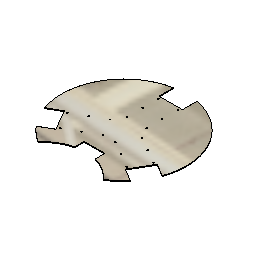
BaseChapaBaixo (Autodesk Fusion 360 design; units mm, degrees)
Autodesk Fusion 360 part; units mm, degrees
note: some values were not read from the file. Set by a fixed rule: which sketch regions a step uses.
sketch "Sketch1" plane through (0, 0, 0) normal (0, 1, 0) x (1, 0, 0)
  circle A0 centre (0, 0) radius 240
  line L0 (0, 0) -> (-207.8461, -120)
  line L1 (0, 0) -> (240, 0) construction
  line L2 (0, 0) -> (207.8461, -120)
  line L3 (0, 0) -> (240, 0) construction
  line L4 (0, 0) -> (0, 240)
  line L5 (0, 240) -> (0, 180)
  line L6 (0, 180) -> (-45, 180)
  line L7 (0, 180) -> (45, 180)
  line L8 (45, 180) -> (45, 235.7435)
  line L9 (-45, 180) -> (-45, 179.9979)
  line L10 (-45, 179.9979) -> (-45, 235.7435)
  line L11 (-133.3828, -128.9701) -> (-181.6599, -156.8429)
  line L12 (-155.8846, -90) -> (-133.3846, -128.9711)
  line L13 (-155.8846, -90) -> (-178.3846, -51.0289)
  line L14 (-178.3846, -51.0289) -> (-226.6599, -78.9006)
  line L15 (178.3828, -51.0278) -> (226.6599, -78.9006)
  line L16 (155.8846, -90) -> (178.3846, -51.0289)
  line L17 (155.8846, -90) -> (133.3846, -128.9711)
  line L18 (133.3846, -128.9711) -> (181.6599, -156.8429)
  line L19 (0, 180) -> (-37.5, 180)
  line L20 (-37.5, 180) -> (-37.5, 169.5)
  circle A1 centre (-37.5, 169.5) radius 2.5
  line L21 (-37.5, 169.5) -> (-37.5, 109.5)
  line L22 (-37.5, 109.5) -> (-37.5, 49.5)
  circle A2 centre (-37.5, 109.5) radius 2.5
  circle A3 centre (-37.5, 49.5) radius 2.5
  line L23 (37.5, 109.5) -> (37.5, 49.5)
  circle A4 centre (37.5, 49.5) radius 2.5
  circle A5 centre (37.5, 109.5) radius 2.5
  line L24 (37.5, 169.5) -> (37.5, 109.5)
  circle A6 centre (37.5, 169.5) radius 2.5
  line L25 (37.5, 180) -> (37.5, 169.5)
  circle A7 centre (-165.5413, -52.274) radius 2.5
  circle A8 centre (-113.5798, -22.274) radius 2.5
  circle A9 centre (-61.6183, 7.726) radius 2.5
  circle A10 centre (-24.1183, -57.226) radius 2.5
  circle A11 centre (-76.0798, -87.226) radius 2.5
  circle A12 centre (-128.0413, -117.226) radius 2.5
  circle A13 centre (128.0413, -117.226) radius 2.5
  circle A14 centre (76.0798, -87.226) radius 2.5
  circle A15 centre (24.1183, -57.226) radius 2.5
  circle A16 centre (61.6183, 7.726) radius 2.5
  circle A17 centre (113.5798, -22.274) radius 2.5
  circle A18 centre (165.5413, -52.274) radius 2.5
  arc A19 (125.0048, -204.8751) -> (-125.0048, -204.8751) centre (0, -310.93) ccw
  line L26 (-38.4014, -152.3633) -> (-38.4014, -115.0053)
  line L27 (-38.4014, -115.0053) -> (41.5986, -115.0053)
  line L28 (41.5986, -115.0053) -> (41.5986, -152.3633)
  dimension "d90" = 480
  dimension "d91" = 150
  dimension "d92" = 30
  dimension "d100" = 60
  dimension "d101" = 45
  dimension "d102" = 45
  dimension "d104" = 360
  dimension "d105" = 37.5
  dimension "d106" = 10.5
  dimension "d107" = 5
  dimension "d108" = 60
  dimension "d109" = 60
  dimension "d110" = 5
  dimension "d111" = 5
  dimension "d113" = 360
  constraint coincident A0.centre L0.start
  constraint horizontal L1
  constraint horizontal L3
  constraint coincident A0 L4.end
  constraint perpendicular L1 L4
  constraint parallel L4 L5
  constraint perpendicular L5 L6
  constraint perpendicular L5 L7
  constraint coincident A0 L8.end
  constraint perpendicular L7 L8
  constraint perpendicular L6 L9
  constraint coincident A0 L10.end
  constraint perpendicular L6 L10
  constraint perpendicular L5 L19
  constraint perpendicular L6 L20
  constraint coincident L20.end A1.centre
  constraint parallel L20 L21
  constraint parallel L21 L22
  constraint coincident L21.end L22.start
  constraint coincident L22.end A3.centre
  constraint symmetric L4 L19.end L25.start
  constraint symmetric L4 L20.end L24.start
  constraint symmetric L4 A1 A6
  constraint symmetric L4 L21.end L23.start
  constraint symmetric L4 L22.end L23.end
  constraint symmetric L4 A2 A5
  constraint symmetric L4 A3 A4
  constraint vertical L26
  constraint horizontal L27
  constraint vertical L28
  measures "d90" diameter of A0
  measures "d91" angle of L0 L1
  measures "d92" angle of L2 L3
  measures "d100" distance of L4.end L5.end
  measures "d101" distance of L5.end L6.end
  measures "d102" distance of L5.end L7.end
  measures "d105" distance of L5.end L19.end
  measures "d106" distance of L19.end L20.end
  measures "d107" diameter of A1
  measures "d108" distance of L20.end L21.end
  measures "d109" distance of L21.end L22.end
  measures "d110" diameter of A2
  measures "d111" diameter of A3
extrude "Extrude2" add sketch "Sketch1" along normal blind 3 contours A0 L2 L4 L7 L8 L15 L16 | A0 L0 L4 L6 L10 L13 L14 L19 | A0 L0 L2 L11 L12 L17 L18 A19 L26 L27 L28
equation "d92 = 150 deg - 120 deg"
equation "d101 = ( 90 / 2 ) * 1 mm"
equation "d102 = ( 90 / 2 ) * 1 mm"
equation "d61 = ( 42 / 2 ) * 1 mm"
